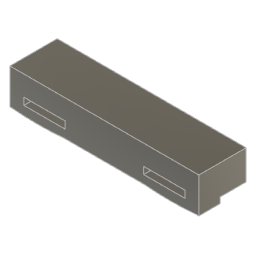
belt holder (Autodesk Fusion 360 design; units mm, degrees)
Autodesk Fusion 360 part; units mm, degrees
note: some values were not read from the file. Chosen so that the rebuilt part matches the saved one: which face or edge a step refers to. Set by a fixed rule: which sketch regions a step uses.
sketch "Sketch1" plane through (0, 0, 0) normal (0, 1, 0) x (1, 0, 0)
  line L0 (0, 0) -> (80, 0)
  line L1 (80, 0) -> (80, -15)
  line L2 (80, -15) -> (0, -15)
  line L3 (0, -15) -> (0, 0)
  dimension "d1" = 80
  dimension "d2" = 15
  constraint horizontal L0
  constraint vertical L1
  constraint horizontal L2
  constraint vertical L3
  constraint coincident L0.start L3.end
  measures "d1" distance of L0.start L0.end
  measures "d2" distance of L0.start L2.end
extrude "Extrude1" add sketch "Sketch1" along normal blind 20
sketch "Sketch2" plane through (0, 0, 0) normal (0, -1, 0) x (1, 0, 0)
  line L0 (80, 15) -> (0, 15)
  line L1 (0, 15) -> (0, 0)
  line L2 (0, 0) -> (80, 0)
  line L3 (80, 0) -> (80, 15)
  line L4 (40, 15) -> (40, 0) construction
  line L5 (5.875, 6.5) -> (23.375, 6.5)
  line L6 (23.375, 6.5) -> (23.375, 3.5)
  line L7 (23.375, 3.5) -> (5.875, 3.5)
  line L8 (5.875, 3.5) -> (5.875, 6.5)
  line L9 (74.125, 6.5) -> (56.625, 6.5)
  line L10 (74.125, 3.5) -> (74.125, 6.5)
  line L11 (56.625, 3.5) -> (74.125, 3.5)
  line L12 (56.625, 6.5) -> (56.625, 3.5)
  dimension "d5" = 17.5
  dimension "d6" = 3
  dimension "d7" = 16.625
  dimension "d8" = 3.5
  constraint midpoint L0 L4.start
  constraint midpoint L2 L4.end
  constraint horizontal L5
  constraint vertical L6
  constraint horizontal L7
  constraint vertical L8
  constraint symmetric L4 L5.start L9.start
  constraint symmetric L4 L5.end L9.end
  constraint symmetric L4 L6.end L11.start
  constraint symmetric L4 L7.end L10.start
  measures "d5" distance of L5.start L5.end
  measures "d6" distance of L5.start L7.end
  measures "d7" distance of L4 L6
  measures "d8" distance of L2 L7
extrude "Extrude2" cut sketch "Sketch2" against normal blind 6.1 contours L5 L6 L7 L8 | L9 L10 L11 L12
sketch "Sketch3" plane through (0, 20, 0) normal (0, 1, 0) x (-1, 0, 0)
  line L0 (0, 15) -> (-80, 15)
  line L1 (-80, 15) -> (-80, 0)
  line L2 (-80, 0) -> (0, 0)
  line L3 (0, 0) -> (0, 15)
  line L4 (-40, 15) -> (-40, 0) construction
  line L5 (0, 7.2533) -> (-80, 7.2533) construction
  circle A0 centre (-55, 7.2533) radius 6
  circle A1 centre (-55, 7.2533) radius 4.25
  line L6 (-54.6901, 1.2613) -> (-79.08, 0)
  line L7 (-80, 2.4558) -> (-72.0811, 2.8653)
  line L8 (-65.8549, 5.4671) -> (-59.0456, 11.6843)
  arc A2 (-72.0811, 2.8653) -> (-65.8549, 5.4671) centre (-72.5976, 12.8519) ccw
  circle A3 centre (-25, 7.2533) radius 4.25
  circle A4 centre (-25, 7.2533) radius 6
  line L9 (-14.1451, 5.4671) -> (-20.9544, 11.6843)
  line L10 (-25.3099, 1.2613) -> (-0.92, 0)
  line L11 (0, 2.4558) -> (-7.9189, 2.8653)
  arc A5 (-14.1451, 5.4671) -> (-7.9189, 2.8653) centre (-7.4024, 12.8519) ccw
  arc A6 (-79.08, 0) -> (-57.08, 0) centre (-68.08, 120.75) ccw
  arc A7 (-22.92, 0) -> (-0.92, 0) centre (-11.92, 120.75) ccw
  arc A8 (-75.5165, 0.1843) -> (-76.3808, -0.2155) centre (-75.4505, -1.0924) ccw
  arc A9 (-3.6192, -0.2155) -> (-4.4835, 0.1843) centre (-4.5495, -1.0924) ccw
  line L12 (-30.4853, 4.7533) -> (-49.5147, 4.7533)
  line L13 (-49.5147, 4.7533) -> (-49.5147, 9.7533)
  line L14 (-49.5147, 9.7533) -> (-30.4853, 9.7533)
  line L15 (-30.4853, 9.7533) -> (-30.4853, 4.7533)
  line L16 (-30.4853, 4.7533) -> (-49.5147, 9.7533) construction
  line L17 (-49.5147, 4.7533) -> (-30.4853, 9.7533) construction
  point P0 (-40, 7.2533)
  dimension "d17" = 8.5
  dimension "d18" = 2.5
  dimension "d20" = 12
  dimension "d21" = 10
  dimension "d22" = 0.5
  dimension "d25" = 22
  dimension "d26" = 15
  dimension "d27" = 5
  constraint midpoint L0 L4.start
  constraint midpoint L2 L4.end
  constraint horizontal L5
  constraint coincident L1 L5.end
  constraint coincident L3 L5.start
  constraint coincident L5 A0.centre
  constraint concentric A0 A1
  constraint coincident A0 L6.start
  constraint coincident L2 L6.end
  constraint tangent A0 L6
  constraint coincident L1 L7.start
  constraint parallel L6 L7
  constraint coincident A0 L8.end
  constraint tangent A0 L8
  constraint tangent L8 A2
  constraint tangent L7 A2
  constraint symmetric L4 A0 A4
  constraint symmetric L4 A1 A3
  constraint symmetric L4 L6.start L10.start
  constraint symmetric L4 L6.end L10.end
  constraint symmetric L4 L7.start L11.start
  constraint symmetric L4 L8.end L9.end
  constraint symmetric L4 L8.start L9.start
  constraint symmetric L4 L7.end L11.end
  constraint symmetric L4 A2 A5
  constraint coincident L2 A6.end
  constraint symmetric L4 A6.end A7.start
  constraint symmetric L4 A6 A7
  constraint tangent L6 A8
  constraint coincident A6 A8.end
  constraint coincident L6 A8.start
  constraint symmetric L4 A8.start A9.end
  constraint symmetric L4 A8.end A9.start
  constraint symmetric L4 A8 A9
  constraint horizontal L12
  constraint perpendicular L12 L13
  constraint parallel L12 L14
  constraint parallel L13 L15
  constraint coincident L16 P0
  constraint coincident L17 P0
  constraint midpoint L5 P0
  measures "d17" diameter of A1
  measures "d18" distance of L6 L7
  measures "d20" diameter of A0
  measures "d21" radius of A2
  measures "d22" distance of L2 A6
  measures "d25" distance of L6.end A6.end
  measures "d26" distance of L4 A0.centre
  measures "d27" distance of L12.end L13.end
extrude "Extrude4" add sketch "Sketch3" against normal blind 20 contours L2 A7 A9 | L2 L6 A8 | L2 A6 A8 | L2 A7 A9 | L2 A6 A8
extrude "Extrude3" cut sketch "Sketch3" against normal blind 11 contours L2 L3 A4 L9 L10 L11 A5 | L1 L2 A0 L6 L7 L8 A2 | L2 A7 A9 | L2 L10 A9 | L2 L6 A8 | L2 A6 A8 | A4 L15 | A0 L13 | A4 L15 | A0 A4 L12 L13 L14 L15 | A0 L13 picked at (-2.8079, -0.0763) picked at (-77.1921, -0.0763)
sketch "Sketch4" plane through (0, 9, 0) normal (0, 1, 0) x (-1, 0, 0)
  circle A0 centre (-55, 7.2533) radius 4.25
  circle A1 centre (-25, 7.2533) radius 4.25
  arc A2 (-49.5147, 9.6847) -> (-59.0456, 11.6843) centre (-55, 7.2533) ccw
  line L0 (-59.0456, 11.6843) -> (-65.8549, 5.4671)
  arc A3 (-72.0811, 2.8653) -> (-65.8549, 5.4671) centre (-72.5976, 12.8519) ccw
  line L1 (-72.0811, 2.8653) -> (-80, 2.4558)
  line L2 (-80, 2.4558) -> (-80, 0)
  line L3 (-80, 0) -> (-79.08, 0)
  arc A4 (-79.08, 0) -> (-76.3808, -0.2155) centre (-68.08, 120.75) ccw
  arc A5 (-75.5165, 0.1843) -> (-76.3808, -0.2155) centre (-75.4505, -1.0924) ccw
  line L4 (-75.5165, 0.1843) -> (-54.6901, 1.2613)
  arc A6 (-54.6901, 1.2613) -> (-49.5147, 4.822) centre (-55, 7.2533) ccw
  line L5 (-49.5147, 4.822) -> (-49.5147, 4.7533)
  line L6 (-49.5147, 4.7533) -> (-30.4853, 4.7533)
  line L7 (-30.4853, 4.7533) -> (-30.4853, 4.822)
  arc A7 (-30.4853, 4.822) -> (-25.3099, 1.2613) centre (-25, 7.2533) ccw
  line L8 (-25.3099, 1.2613) -> (-4.4835, 0.1843)
  arc A8 (-3.6192, -0.2155) -> (-4.4835, 0.1843) centre (-4.5495, -1.0924) ccw
  arc A9 (-3.6192, -0.2155) -> (-0.92, 0) centre (-11.92, 120.75) ccw
  line L9 (-0.92, 0) -> (0, 0)
  line L10 (0, 0) -> (0, 2.4558)
  line L11 (0, 2.4558) -> (-7.9189, 2.8653)
  arc A10 (-14.1451, 5.4671) -> (-7.9189, 2.8653) centre (-7.4024, 12.8519) ccw
  line L12 (-14.1451, 5.4671) -> (-20.9544, 11.6843)
  arc A11 (-20.9544, 11.6843) -> (-30.4853, 9.6847) centre (-25, 7.2533) ccw
  line L13 (-30.4853, 9.6847) -> (-30.4853, 9.7533)
  line L14 (-30.4853, 9.7533) -> (-49.5147, 9.7533)
  line L15 (-49.5147, 9.7533) -> (-49.5147, 9.6847)
  line L16 (-49.5147, 9.7533) -> (-51.5631, 9.7533)
  line L17 (-51.5631, 9.7533) -> (-51.5631, 4.7236)
  line L18 (-51.5631, 4.7236) -> (-49.5147, 4.7236)
  line L19 (-49.5147, 4.7236) -> (-49.5147, 9.7533)
  line L20 (0, 15) -> (-80, 15) construction
  line L21 (-40, 15) -> (-40, 0) construction
  line L22 (-30.4853, 9.7533) -> (-28.4369, 9.7533)
  line L23 (-28.4369, 9.7533) -> (-28.4369, 4.7236)
  line L24 (-28.4369, 4.7236) -> (-30.4853, 4.7236)
  line L25 (-30.4853, 4.7236) -> (-30.4853, 9.7533)
  constraint perpendicular L16 L17
  constraint parallel L16 L18
  constraint parallel L17 L19
  constraint coincident A0 L16.end
  constraint perpendicular L15 L16
  constraint coincident L14.end L15.start
  constraint midpoint L20 L21.start
  constraint perpendicular L20 L21
  constraint symmetric L14.end L21 L13.end
  constraint symmetric L16.end L21 L22.end
  constraint symmetric L17.end L21 L23.end
  constraint symmetric L18.end L21 L24.end
extrude "Extrude5" [rolled back] along distance -2 taper angle 0
fillet "Fillet1" [rolled back] radius 1.5 radius 1.5
sketch "Sketch5" plane through (0, 20, 0) normal (0, 1, 0) x (-1, 0, 0)
  line L0 (-80, 2.4558) -> (-72.0811, 2.8653)
  arc A0 (-72.0811, 2.8653) -> (-65.8549, 5.4671) centre (-72.5976, 12.8519) ccw
  line L1 (-65.8549, 5.4671) -> (-59.0456, 11.6843)
  arc A1 (-49.5147, 9.6847) -> (-59.0456, 11.6843) centre (-55, 7.2533) ccw
  line L2 (-49.5147, 9.6847) -> (-49.5147, 9.7533)
  line L3 (-49.5147, 9.7533) -> (-30.4853, 9.7533)
  line L4 (-30.4853, 9.7533) -> (-30.4853, 9.6847)
  arc A2 (-20.9544, 11.6843) -> (-30.4853, 9.6847) centre (-25, 7.2533) ccw
  line L5 (-20.9544, 11.6843) -> (-14.1451, 5.4671)
  arc A3 (-14.1451, 5.4671) -> (-7.9189, 2.8653) centre (-7.4024, 12.8519) ccw
  line L6 (-7.9189, 2.8653) -> (0, 2.4558)
  line L7 (0, 2.4558) -> (0, 15)
  line L8 (0, 15) -> (-80, 15)
  line L9 (-80, 15) -> (-80, 2.4558)
  arc A4 (-75.5165, 0.1843) -> (-76.3808, -0.2155) centre (-75.4505, -1.0924) ccw
  arc A5 (-76.3808, -0.2155) -> (-57.08, 0) centre (-68.08, 120.75) ccw
  line L10 (-57.08, 0) -> (-22.92, 0)
  arc A6 (-22.92, 0) -> (-3.6192, -0.2155) centre (-11.92, 120.75) ccw
  arc A7 (-3.6192, -0.2155) -> (-4.4835, 0.1843) centre (-4.5495, -1.0924) ccw
  line L11 (-4.4835, 0.1843) -> (-25.3099, 1.2613)
  arc A8 (-30.4853, 4.822) -> (-25.3099, 1.2613) centre (-25, 7.2533) ccw
  line L12 (-30.4853, 4.822) -> (-30.4853, 4.7533)
  line L13 (-30.4853, 4.7533) -> (-49.5147, 4.7533)
  line L14 (-49.5147, 4.7533) -> (-49.5147, 4.822)
  arc A9 (-54.6901, 1.2613) -> (-49.5147, 4.822) centre (-55, 7.2533) ccw
  line L15 (-54.6901, 1.2613) -> (-75.5165, 0.1843)
  line L16 (-76.3808, -0.2155) -> (-76.3808, 2.6429) construction
  line L17 (-76.3808, 2.6429) -> (-76.3808, 4.6429)
  line L18 (-71.3808, -0.4551) -> (-71.3808, 2.9263)
  line L19 (-71.3808, 4.6429) -> (-71.3808, 2.9263)
  line L20 (-71.3808, 4.6429) -> (-76.3808, 4.6429)
  line L21 (-40, 15) -> (-40, 0) construction
  line L22 (-8.6192, 4.6429) -> (-3.6192, 4.6429)
  line L23 (-3.6192, 2.6429) -> (-3.6192, 4.6429)
  line L24 (-8.6192, 4.6429) -> (-8.6192, 2.9263)
  line L25 (-8.6192, -0.4551) -> (-8.6192, 2.9263)
  line L26 (-3.6192, -0.2155) -> (-3.6192, 2.6429) construction
  dimension "d34" = 2
  dimension "d35" = 5
  constraint coincident A4.end A5.start
  constraint coincident L0 L16.end
  constraint vertical L16
  constraint vertical L17
  constraint coincident A5 L18.start
  constraint coincident A0 L18.end
  constraint parallel L17 L18
  constraint parallel L18 L19
  constraint perpendicular L17 L20
  constraint midpoint L8 L21.start
  constraint midpoint L10 L21.end
  constraint symmetric A4.end L21 A6.end
  constraint symmetric L16.end L21 L23.start
  constraint symmetric L17.end L21 L22.end
  constraint symmetric L18.start L21 L25.start
  constraint symmetric L18.end L21 L24.end
  constraint symmetric L19.start L21 L22.start
  measures "d34" distance of L16.end L17.end
  measures "d35" distance of L17.end L19.start
extrude "Extrude6" [rolled back] along distance 7.5 taper angle 0
sketch "Sketch6" plane through (0, 0, 4.6429) normal (0, 0, 1) x (-1, 0, 0)
  line L0 (-71.3808, -20) -> (-76.3808, -20)
  line L1 (-76.3808, -20) -> (-76.3808, -27.5)
  line L2 (-76.3808, -27.5) -> (-71.3808, -27.5)
  line L3 (-71.3808, -27.5) -> (-71.3808, -20)
  line L4 (-76.3808, -27.5) -> (-71.3808, -27.5)
  line L5 (-71.3808, -27.5) -> (-71.3808, -25.5)
  line L6 (-71.3808, -25.5) -> (-76.3808, -25.5)
  line L7 (-76.3808, -25.5) -> (-76.3808, -27.5)
  dimension "d38" = 2
  constraint horizontal L4
  constraint vertical L5
  constraint horizontal L6
  constraint vertical L7
  constraint coincident L1.end L2.start
  measures "d38" distance of L1.end L6.end
extrude "Extrude7" [rolled back] side1offset 0 taper angle 0
fillet "Fillet2" [rolled back] radius 1
ref_plane "WorkPlane1" through (40, 10, 7.5) normal (1, 0, 0) x (0, 0, -1)
mirror "Mirror1" [rolled back] mirror stitch tolerance 0.1
mirror "Mirror2" [rolled back] mirror stitch tolerance 0.1
chamfer "Chamfer1" [rolled back] distance 6
equation "d7 = ( 33.25 / 2 ) * 1 mm"
